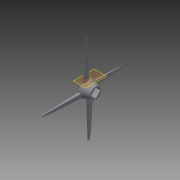
# Autodesk Inventor part: Нож
Saved by Autodesk Inventor 2014 SP1 (Build 180222100, 222)
## iProperties
Created: 2023-07-18
Part Number: Нож
Material: Типовые
Document SubType Name: Modeling
Designer: 1.507-7
Density: 1 g/cm^3
Appearance: По умолчанию
Author: 1.507-7
Autodesk Inventor part; units mm, degrees
ref_plane "YZ Plane" through (0, 0, 0) normal (1, 0, 0) x (0, 1, 0)
ref_plane "XZ Plane" through (0, 0, 0) normal (0, 1, 0) x (-1, 0, 0)
ref_plane "XY Plane" through (0, 0, 0) normal (0, 0, 1) x (1, 0, 0)
sketch "Эскиз1" plane through (0, 0, 0) normal (1, 0, 0) x (0, 1, 0)
  circle A0 centre (0, 0) radius 5
  line L0 (0, -2.5) -> (2.5037, 0)
  line L1 (2.5037, 0) -> (0, 2.5074)
  line L2 (0, 2.5074) -> (-2.5037, 0.0074)
  line L3 (-2.5037, 0.0074) -> (0, -2.5)
  constraints: 8 end point, 2 parallel, 1 centre point, 1 coincident, 1 perpendicular
extrude "Выдавливание1" add sketch "Эскиз1" along normal blind 6
chamfer "Фаска1" distance 6 distance2 2 1 edges at (6, -5, 0) measured on face at (4, 4.9353, -0.8021)
ref_plane "РабПлоскость3" through (0, 0, 5.25) normal (0, 0, 1) x (1, 0, 0)
sketch "Эскиз5" plane through (0, 0, 5.25) normal (0, 0, 1) x (1, 0, 0)
  line L0 (0, 1) -> (2.4, 0)
  line L1 (2.4, 0) -> (2.4, -2)
  line L2 (2.4, -2) -> (1.6636, -2.3125)
  line L3 (0, 1) -> (1.6636, -2.3125)
  point P0 (0, 0)
  constraints: 8 end point, 1 vertical
extrude "Выдавливание2" add sketch "Эскиз5" along normal blind 19 draft -2 and the other way blind 2
pattern_circular "Круговой массив1" count 4 over 360 about axis through (3, 0, 0) along (1, 0, 0) of "Выдавливание2"
sketch "Эскиз6" plane through (0, 0, 0) normal (0, 1, 0) x (-1, 0, 0)
  line L0 (-1.1407, -15.27) -> (6.3977, -15.27)
  line L1 (6.3977, -15.27) -> (6.3977, 15.5226)
  line L2 (6.3977, 15.5226) -> (-1.1407, 15.5226)
  line L3 (-1.1407, 15.5226) -> (-1.1407, -15.27)
  point P0 (0, 0)
  constraints: 8 end point, 2 parallel, 1 horizontal, 1 perpendicular
extrude "Выдавливание3" cut sketch "Эскиз6" along normal through all both and the other way through all
sketch "Эскиз7" plane through (0, 0, 0) normal (0, 1, 0) x (-1, 0, 0)
  line L0 (-1.4062, -24.2443) -> (6.1599, -24.2443)
  line L1 (6.1599, -24.2443) -> (6.1599, 24.4007)
  line L2 (6.1599, 24.4007) -> (-1.4062, 24.4007)
  line L3 (-1.4062, 24.4007) -> (-1.4062, -24.2443)
  point P0 (0, 0)
  constraints: 8 end point, 2 parallel, 1 horizontal, 1 perpendicular
extrude "Выдавливание4" cut sketch "Эскиз7" along normal through all both and the other way through all
